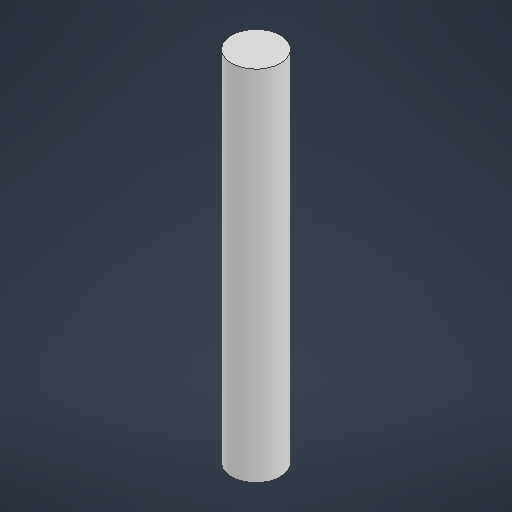
# Autodesk Inventor part: eixo 4
Saved by Autodesk Inventor 2026.2 (Build 302298000, 298)
## iProperties
Created: 2026-09-11
Part Number: eixo 4
Material: Genérico
Document SubType Name: Modeling
Designer: IFSP
Density: 1 g/cm^3
Appearance: Padrão
Author: IFSP
Autodesk Inventor part; units mm, degrees
sketch "Esboço1" plane through (0, 0, 0) normal (0, 1, 0) x (-1, 0, 0)
  circle A0 centre (0, 0) radius 6
  dimension "d0" = 12
  constraints: 1 centre point, 1 coincident
  measures "d0" diameter of A0
extrude "Extrusão1" add sketch "Esboço1" along normal blind 88
ref_plane "Plano de trabalho1" through (0, 0, -6) normal (0, 0, 1) x (1, 0, 0)
ref_plane "Plano de trabalho2" through (0, 0, -6) normal (0, 0, 1) x (1, 0, 0)
ref_plane "Plano de trabalho3" through (0, 0, 6) normal (0, 0, 1) x (1, 0, 0)
sketch "Esboço2" plane through (0, 0, -6) normal (0, 0, 1) x (1, 0, 0)
  line L0 (0, 92.3715) -> (0, -4.0857) construction
  line L1 (-6, 0) -> (-6, 88) construction
  line L2 (-6, 88) -> (-6, 58) construction
  line L3 (-6, 58) -> (-6, 48) construction
  line L4 (0, 58) -> (0, 48) construction
  line L5 (-1.25, 58) -> (-1.25, 48)
  line L6 (1.25, 48) -> (1.25, 58)
  arc A0 (1.25, 58) -> (-1.25, 58) centre (0, 58) ccw
  arc A1 (-1.25, 48) -> (1.25, 48) centre (0, 48) ccw
  line L7 (-6, 0) -> (-6, 10) construction
  line L8 (0, 10) -> (0, 0) construction
  line L9 (-1.25, 10) -> (-1.25, 0)
  line L10 (1.25, 0) -> (1.25, 10)
  arc A2 (1.25, 10) -> (-1.25, 10) centre (0, 10) ccw
  arc A3 (-1.25, 0) -> (1.25, 0) centre (0, 0) ccw
  point P0 (0, 53)
  point P1 (0, 5)
  dimension "d4" = 30
  dimension "d5" = 10
  dimension "d6" = 2.5
  dimension "d7" = 10
  dimension "d8" = 2.5
  constraints: 24 end point, 8 point on circle, 8 tangent, 7 point on line, 4 centre point, 2 midpoint, 2 parallel, 1 collinear, 1 vertical
  measures "d4" distance of L2.start L2.end
  measures "d5" distance of L2.end L3.end
  measures "d6" diameter of A1
  measures "d7" distance of L1.start L7.end
  measures "d8" diameter of A3
extrude "Extrusão2" cut sketch "Esboço2" along normal blind 2.5
